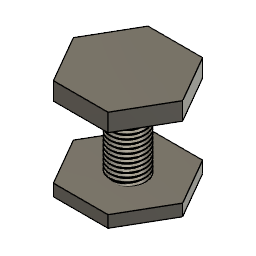
Learning part 2 (Autodesk Fusion 360 design; units mm, degrees)
part number: 2025-11-20-19-16-30-243
part number: 2025-11-20-19-39-59-449
part number: 2025-11-20-19-40-54-755
Autodesk Fusion 360 part; units mm, degrees
sketch "Sketch1" plane through (0, 0, 0) normal (0, 1, 0) x (1, 0, 0)
  line L0 (23.094, -40) -> (46.188, 0)
  line L1 (46.188, 0) -> (23.094, 40)
  line L2 (23.094, 40) -> (-23.094, 40)
  line L3 (-23.094, 40) -> (-46.188, 0)
  line L4 (-46.188, 0) -> (-23.094, -40)
  line L5 (-23.094, -40) -> (23.094, -40)
  dimension "d1" = 40
  measures "d1" distance of origin L5
extrude "Extrude1" add sketch "Sketch1" along normal blind 10 makes body 1
sketch "Sketch2" plane through (0, 10, 0) normal (0, 1, 0) x (-1, 0, 0)
  line L0 (23.094, 40) -> (-23.094, 40)
  line L1 (-23.094, 40) -> (-46.188, 0)
  line L2 (-46.188, 0) -> (-23.094, -40)
  line L3 (-23.094, -40) -> (23.094, -40)
  line L4 (23.094, -40) -> (46.188, 0)
  line L5 (46.188, 0) -> (23.094, 40)
  circle A0 centre (0, 0) radius 10
  dimension "d4" = 20
  constraint coincident A0.centre origin
  measures "d4" diameter of A0
extrude "Extrude2" cut sketch "Sketch2" against normal up to surface (10 mm away) contours A0 bodies 1
thread "Thread1" "ISO Metric profile 28.0 M28x2 M28x2 6H" major diameter 28.2565 minor diameter 26.0224 pitch 2 angle 60 resizes the face on face at (-9.9876, 3.3333, -0.4985) on bodies 1
copy_body "Body->Comp1" bodies 1 removing the originals makes body 2 in component "nut"
sketch "Sketch1 (2)" plane through (0, 0, 0) normal (0, 1, 0) x (1, 0, 0) in component "Bolt"
  circle A0 centre (0, 0) radius 10
  dimension "d9" = 20
  constraint coincident A0.centre origin
  measures "d9" diameter of A0
extrude "Extrude1'" add sketch "Sketch1 (2)" along normal blind 70 separate body makes body 3 in component "Bolt"
sketch "Sketch2 (2)" plane through (0, 70, 0) normal (0, 1, 0) x (-1, 0, 0) in component "Bolt"
  circle A0 centre (0, 0) radius 10
  line L0 (-23.094, 40) -> (-46.188, 0)
  line L1 (-46.188, 0) -> (-23.094, -40)
  line L2 (-23.094, -40) -> (23.094, -40)
  line L3 (23.094, -40) -> (46.188, 0)
  line L4 (46.188, 0) -> (23.094, 40)
  line L5 (23.094, 40) -> (-23.094, 40)
  constraint coincident A0.centre origin
extrude "Extrude2'" add sketch "Sketch2 (2)" along normal blind 15 contours A0 | L0 L1 L2 L3 L4 L5 bodies 3 in component "Bolt"
thread "Thread1'" "ISO Metric profile 30.0 M30x3.5 M30x3.5 6g" major diameter 29.7345 minor diameter 25.732 pitch 3.5 angle 60 modelled right hand crest width 0.4992 on face at (9.9503, 46.6667, 0.9957) crest through (14.8673, -0.875, 0) on bodies 3 in component "Bolt"
thread "Thread1''" "ISO Metric profile 30.0 M30x3.5 M30x3.5 6H" major diameter 30.3925 minor diameter 26.491 pitch 3.5 angle 60 resizes the face on face at (-12.995, 3.3333, -0.6486) on bodies 2 in component "nut"
component "nut" placed x (1, 0, 0) y (0, 1, 0) z (0, 0, 1) at (0, 0, 0)
component "Bolt" placed x (1, 0, 0) y (0, 1, 0) z (0, 0, 1) at (0, 0, 0)
named bodies: "nut"
